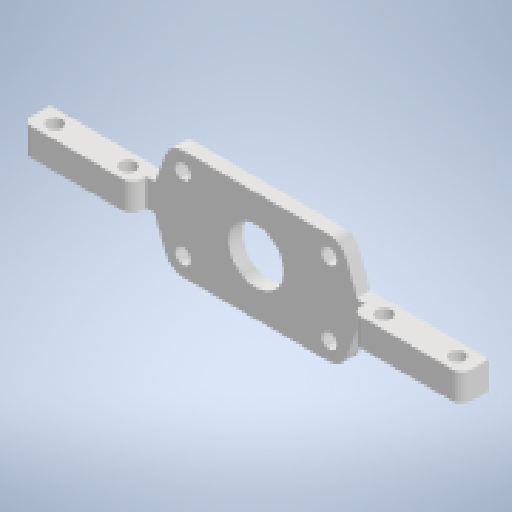
# Autodesk Inventor part: Face Plate
Saved by Autodesk Inventor 2023 (Build 270158000, 158)
## iProperties
Created: 2023-02-27
Part Number: Face Plate
Material: Generic
Document SubType Name: Modeling
Designer: Gabriel - T3 CAD
Density: 1 g/cm^3
Appearance: Default
Author: Gabriel - T3 CAD
Autodesk Inventor part; units mm, degrees
ref_plane "YZ Plane" through (0, 0, 0) normal (1, 0, 0) x (0, 1, 0)
ref_plane "XZ Plane" through (0, 0, 0) normal (0, 1, 0) x (-1, 0, 0)
ref_plane "XY Plane" through (0, 0, 0) normal (0, 0, 1) x (1, 0, 0)
sketch "Sketch1" plane through (0, 0, 0) normal (0, 1, 0) x (-1, 0, 0)
  line L0 (0, 0) -> (152.4, 0)
  line L1 (152.4, 0) -> (152.4, 6.35)
  line L2 (34.925, 9.525) -> (3.175, 9.525)
  line L3 (0, 6.35) -> (0, 0)
  circle A0 centre (6.35, 4.7625) radius 2.5797
  circle A1 centre (31.75, 4.7625) radius 2.5797
  circle A2 centre (120.65, 4.7625) radius 2.5797
  circle A3 centre (146.05, 4.7625) radius 2.5797
  line L4 (38.1, 9.525) -> (114.3, 9.525)
  line L5 (114.3, 6.35) -> (114.3, 4.7625)
  line L6 (114.3, 4.7625) -> (38.1, 4.7625)
  line L7 (38.1, 4.7625) -> (38.1, 6.35)
  arc A4 (38.1, 6.35) -> (34.925, 9.525) centre (34.925, 6.35) ccw
  arc A5 (3.175, 9.525) -> (0, 6.35) centre (3.175, 6.35) ccw
  line L8 (117.475, 9.525) -> (149.225, 9.525)
  arc A6 (117.475, 9.525) -> (114.3, 6.35) centre (117.475, 6.35) ccw
  arc A7 (152.4, 6.35) -> (149.225, 9.525) centre (149.225, 6.35) ccw
  line L9 (114.3, 6.35) -> (114.3, 0)
  line L10 (38.1, 6.35) -> (38.1, 0)
  line L11 (114.3, 4.7625) -> (114.3, 9.525)
  line L12 (117.475, 9.525) -> (114.3, 9.525)
  line L13 (38.1, 6.35) -> (38.1, 9.525)
  line L14 (38.1, 9.525) -> (34.925, 9.525)
  point P0 (152.4, 9.525)
  point P1 (0, 9.525)
  point P2 (38.1, 4.7625)
  dimension "d0" = 152.4
  dimension "d1" = 9.525
  dimension "d2" = 4.7625
  dimension "d3" = 4.7625
  dimension "d4" = 4.7625
  dimension "d5" = 4.7625
  dimension "d6" = 25.4
  dimension "d7" = 25.4
  dimension "d8" = 5.1594
  dimension "d9" = 6.35
  dimension "d10" = 6.35
  dimension "d11" = 4.7625
  dimension "d12" = 6.35
  dimension "d13" = 6.35
  dimension "d14" = 3.175
  dimension "d15" = 3.175
  constraints: 30 end point, 11 point on line, 10 tangent, 8 centre point, 8 point on circle, 7 perpendicular, 5 equal radius, 4 parallel, 2 horizontal
  measures "d0" distance of point (152.4, 9.525) point (0, 9.525)
  measures "d1" distance of L0.end point (152.4, 9.525)
  measures "d2" distance from line of L0 A0.centre
  measures "d3" distance from line of L0 A1.centre
  measures "d4" distance from line of L0 A2.centre
  measures "d5" distance from line of L0 A3.centre
  measures "d6" distance of A0.centre A1.centre
  measures "d7" distance of A2.centre A3.centre
  measures "d8" diameter of A3
  measures "d9" distance from line of L3 A0.centre
  measures "d10" distance from line of L1 A3.centre
  measures "d11" distance of L6.end L4.start
  measures "d12" distance from line of A1.centre L7
  measures "d13" distance from line of A2.centre L5
  measures "d14" radius of A4
  measures "d15" radius of A6
extrude "Extrusion1" add sketch "Sketch1" along normal mid plane 9.525 contours L3 A5 L2 A4 L7 L10 L0 | L10 L6 L9 L0 | L9 L5 A6 L8 A7 L1 L0
extrude "Extrusion2" add sketch "Sketch1" along normal mid plane 50.8 contours L10 L6 L9 L0
sketch "Sketch2" plane through (-114.3, 25.4, 4.7625) normal (0, 0, 1) x (1, 0, 0)
  line L0 (76.2, -30.1625) -> (76.2, -50.8) projected
  line L1 (0, 0) -> (76.2, 0)
  line L2 (76.2, 0) -> (76.2, -50.8)
  line L3 (76.2, -50.8) -> (0, -50.8)
  line L4 (0, -50.8) -> (0, 0)
  circle A0 centre (38.1, -25.4) radius 9.525
  line L5 (12.7, -50.8) -> (12.7, 0)
  line L6 (12.7, 0) -> (63.5, 0)
  line L7 (63.5, 0) -> (63.5, -50.8)
  line L8 (63.5, -50.8) -> (12.7, -50.8)
  line L9 (12.7, -12.7) -> (63.5, -12.7)
  line L10 (63.5, -12.7) -> (63.5, -38.1)
  line L11 (63.5, -38.1) -> (12.7, -38.1)
  line L12 (12.7, -38.1) -> (12.7, -12.7)
  circle A1 centre (12.7, -12.7) radius 2.5797
  circle A2 centre (12.7, -38.1) radius 2.5797
  circle A3 centre (63.5, -38.1) radius 2.5797
  circle A4 centre (63.5, -12.7) radius 2.5797
  circle A5 centre (12.7, -12.7) radius 6.35
  circle A6 centre (12.7, -38.1) radius 6.35
  circle A7 centre (63.5, -38.1) radius 6.35
  circle A8 centre (63.5, -12.7) radius 6.35
  line L13 (6.35, -6.35) -> (69.85, -6.35)
  line L14 (69.85, -6.35) -> (69.85, -44.45)
  line L15 (69.85, -44.45) -> (6.35, -44.45)
  line L16 (6.35, -44.45) -> (6.35, -6.35)
  line L17 (0, -20.6375) -> (-3.175, -20.6375) projected
  line L18 (0, -30.1625) -> (0, -20.6375) projected
  line L19 (76.2, -30.1625) -> (76.2, -20.6375) projected
  line L20 (0, -20.6375) -> (6.35, -20.6375)
  line L21 (3.175, -20.6375) -> (12.9069, 7.017)
  line L22 (0, -30.1625) -> (0, -20.6375) projected
  line L23 (0, -30.1625) -> (6.35, -30.1625)
  line L24 (3.175, -30.1625) -> (13.5434, -59.6259)
  line L25 (76.2, -30.1625) -> (69.85, -30.1625)
  line L26 (76.2, -20.6375) -> (76.2, 0) projected
  line L27 (76.2, -20.6375) -> (69.85, -20.6375)
  line L28 (73.025, -20.6375) -> (62.053, 10.5411)
  line L29 (73.025, -30.1625) -> (62.6786, -59.5632)
  point P0 (114.3, -25.4)
  point P1 (63.5, -44.45)
  point P2 (12.7, -44.45)
  point P3 (12.7, -6.35)
  point P4 (63.5, -6.35)
  point P5 (6.35, -38.1)
  point P6 (69.85, -38.1)
  point P7 (69.85, -12.7)
  point P8 (6.35, -12.7)
  point P9 (6.35, -11.6153)
  point P10 (6.7101, -10.5921)
  point P11 (69.4899, -10.5921)
  point P12 (69.4899, -40.2079)
  point P13 (6.7101, -40.2079)
  dimension "d24" = 25.4
  dimension "d25" = 38.1
  dimension "d26" = 50.8
  dimension "d27" = 25.4
  dimension "d28" = 12.7
  dimension "d29" = 19.05
  dimension "d30" = 5.1594
  dimension "d33" = 12.7
  dimension "d34" = 12.7
  dimension "d35" = 12.7
  dimension "d36" = 12.7
  constraints: 48 end point, 10 coincident, 9 centre point, 8 tangent, 7 perpendicular, 6 parallel, 6 point on line, 4 midpoint, 3 equal radius, 3 horizontal, 1 vertical, 9 other
  measures "d24" distance from line of L1 A0.centre
  measures "d25" distance from line of L4 A0.centre
  measures "d26" distance of L5.end L6.end
  measures "d27" distance between parallel lines of L11 L9
  measures "d28" distance between parallel lines of L6 L9
  measures "d29" diameter of A0
  measures "d30" diameter of A1
  measures "d33" diameter of A5
  measures "d34" diameter of A6
  measures "d35" diameter of A7
  measures "d36" diameter of A8
extrude "Extrusion3" cut sketch "Sketch2" against normal through all contours L0 L3 L29 L15 L14 L25 | L27 L28 L14 L13 L1 L2 | L3 L7 L15 L29 | L14 L15 L29 | L3 L5 L15 L7 | L15 A7 L29 | L28 L13 L7 L1 | L28 L13 L14 | L3 L24 L15 L5 | L7 L13 L5 L1 | L28 A8 L13 | L3 L4 L23 L24 L16 L15 | L15 L24 A6 | A3 L11 L7 | L7 A3 | L5 L13 L21 L1 | L7 L11 A3 | L15 L16 L24 | A2 L5 | L5 L11 A2 | L21 L13 L16 L20 L4 L1 | A5 L21 L13 | A4 L7 | L7 L9 A4 | A4 L9 L7 | L5 A2 L11 | L21 L16 L13 | A1 L9 L5 | L5 A1 | L9 A1 L5 | A0
equation "\"d2\" = 0.5 * d1"
equation "\"d3\" = d2"
equation "\"d4\" = d2"
equation "\"d5\" = d2"
equation "\"d10\" = d9"
equation "\"d11\" = 0.5 * d1"
body "Solid1"
